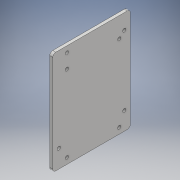
# Autodesk Inventor part: adapter_arduino_to_power
Saved by Autodesk Inventor 2018 (Build 220112000, 112)
## iProperties
Created: 2019-05-08
Part Number: adapter_arduino_to_power
Material: Типовые
Document SubType Name: Modeling
Designer: KV33_HP1
Density: 1 g/cm^3
Appearance: По умолчанию
Author: KV33_HP1
Autodesk Inventor part; units mm, degrees
ref_plane "YZ Plane" through (0, 0, 0) normal (1, 0, 0) x (0, 1, 0)
ref_plane "XZ Plane" through (0, 0, 0) normal (0, 1, 0) x (-1, 0, 0)
ref_plane "XY Plane" through (0, 0, 0) normal (0, 0, 1) x (1, 0, 0)
sketch "Эскиз1" plane through (0, 0, 0) normal (1, 0, 0) x (0, 1, 0)
  circle A0 centre (0, 0) radius 1.65
  circle A1 centre (5, 5) radius 1.65
  circle A2 centre (5, -64) radius 1.65
  circle A3 centre (0, -76) radius 1.65
  circle A4 centre (-52, 14) radius 1.65
  circle A5 centre (-52, 0) radius 1.65
  circle A6 centre (-52, -76) radius 1.65
  circle A7 centre (-60, -64) radius 1.65
  line L0 (-63, 20) -> (8, 20)
  line L1 (11, 17) -> (11, -79)
  line L2 (8, -82) -> (-63, -82)
  line L3 (-66, -79) -> (-66, 17)
  arc A8 (11, 17) -> (8, 20) centre (8, 17) ccw
  arc A9 (8, -82) -> (11, -79) centre (8, -79) ccw
  arc A10 (-66, -79) -> (-63, -82) centre (-63, -79) ccw
  arc A11 (-63, 20) -> (-66, 17) centre (-63, 17) ccw
  dimension "d4" = 3.3
  dimension "d5" = 3.3
  dimension "d7" = 3.3
  dimension "d8" = 3.3
  dimension "d12" = 3.3
  dimension "d13" = 3.3
  dimension "d14" = 3.3
  dimension "d15" = 3.3
  dimension "d20" = 3
  constraints: 12 centre point, 8 end point, 8 point on circle, 8 tangent, 3 equal radius, 2 parallel, 1 coincident, 1 horizontal, 1 perpendicular
  measures "d4" diameter of A0
  measures "d5" diameter of A1
  measures "d7" diameter of A2
  measures "d8" diameter of A3
  measures "d12" diameter of A4
  measures "d13" diameter of A5
  measures "d14" diameter of A6
  measures "d15" diameter of A7
  measures "d20" radius of A8
extrude "Выдавливание1" add sketch "Эскиз1" along normal blind 3
